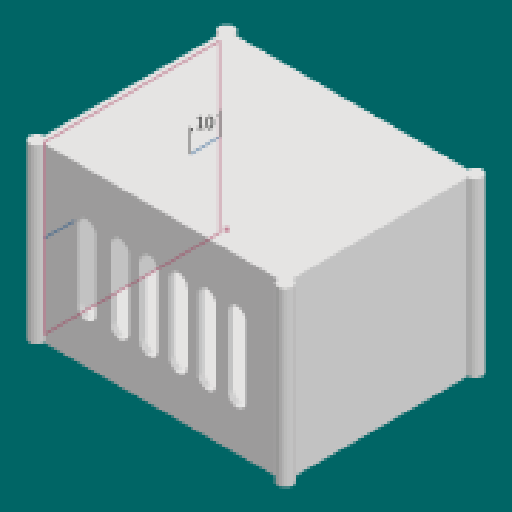
# Autodesk Inventor part: Body_Bottom
Saved by Autodesk Inventor 2025.2 (Build 292293000, 293)
## iProperties
Created: 2025-06-02
Part Number: Body_Bottom
Material: Generic
Document SubType Name: Modeling
Designer: ia088
Density: 1 g/cm^3
Appearance: Default
Author: ia088
Autodesk Inventor part; units mm, degrees
ref_plane "YZ Plane" through (0, 0, 0) normal (1, 0, 0) x (0, 1, 0)
ref_plane "XZ Plane" through (0, 0, 0) normal (0, 1, 0) x (-1, 0, 0)
ref_plane "XY Plane" through (0, 0, 0) normal (0, 0, 1) x (1, 0, 0)
sketch "Sketch1" plane through (0, 0, 0) normal (0, 1, 0) x (-1, 0, 0)
  line L0 (0, 0) -> (-85, 0)
  line L1 (-85, 0) -> (-85, 65)
  line L2 (-85, 65) -> (0, 65)
  line L3 (0, 65) -> (0, 0)
  line L4 (-4, 2) -> (-81, 2)
  line L5 (-83, 4) -> (-83, 61)
  line L6 (-81, 63) -> (-4, 63)
  line L7 (-2, 61) -> (-2, 4)
  circle A0 centre (0, 0) radius 2.5
  circle A1 centre (0, 65) radius 2.5
  circle A2 centre (-85, 65) radius 2.5
  circle A3 centre (-85, 0) radius 2.5
  arc A4 (-4, 2) -> (-2, 4) centre (-4, 4) ccw
  arc A5 (-83, 4) -> (-81, 2) centre (-81, 4) ccw
  arc A6 (-81, 63) -> (-83, 61) centre (-81, 61) ccw
  arc A7 (-2, 61) -> (-4, 63) centre (-4, 61) ccw
  point P0 (0, 62.5)
  point P1 (-2.5, 65)
  point P2 (-82.5, 65)
  point P3 (-85, 62.5)
  point P4 (-85, 2.5)
  point P5 (-82.5, 0)
  point P6 (-2.5, 0)
  point P7 (0, 2.5)
  dimension "d0" = 85
  dimension "d1" = 65
  dimension "d14" = 5
  dimension "d15" = 5
  dimension "d16" = 5
  dimension "d17" = 5
  dimension "d18" = 2
  constraints: 16 end point, 8 centre point, 8 point on circle, 8 tangent, 4 coincident, 4 parallel, 3 equal radius, 2 horizontal, 2 perpendicular
  measures "d0" distance of L1.end L2.end
  measures "d1" distance of L0.end L1.end
  measures "d14" diameter of A0
  measures "d15" diameter of A1
  measures "d16" diameter of A2
  measures "d17" diameter of A3
  measures "d18" radius of A4
extrude "Extrusion1" add sketch "Sketch1" along normal blind 2 contours A3 L1 L0 | A3 L1 A2 L2 A1 L3 A0 L0 | L0 L1 A3 | A0 L3 L0 | L0 L3 A0 | A2 L2 L1 | L1 L2 A2 | A1 L2 L3 | L3 L2 A1 | L4 A5 L5 A6 L6 A7 L7 A4
sketch "Sketch2" plane through (0, 2, 0) normal (0, 1, 0) x (1, 0, 0)
  line L0 (2.5, -65) -> (82.5, -65) projected
  arc A0 (82.5, -65) -> (85, -62.5) centre (85, -65) ccw projected
  line L1 (85, -62.5) -> (85, -2.5) projected
  arc A1 (85, -2.5) -> (82.5, 0) centre (85, 0) ccw projected
  line L2 (82.5, 0) -> (2.5, 0) projected
  arc A2 (2.5, 0) -> (0, -2.5) centre (0, 0) ccw projected
  line L3 (0, -2.5) -> (0, -62.5) projected
  arc A3 (0, -62.5) -> (2.5, -65) centre (0, -65) ccw projected
  line L4 (81, -2) -> (4, -2)
  line L5 (2, -4) -> (2, -61)
  line L6 (4, -63) -> (81, -63)
  line L7 (83, -61) -> (83, -4)
  arc A4 (2, -61) -> (4, -63) centre (4, -61) ccw
  arc A5 (4, -2) -> (2, -4) centre (4, -4) ccw
  arc A6 (81, -63) -> (83, -61) centre (81, -61) ccw
  arc A7 (83, -4) -> (81, -2) centre (81, -4) ccw
  dimension "d25" = 2
  constraints: 8 end point, 8 point on circle, 8 tangent, 4 centre point, 3 equal radius, 2 parallel, 1 horizontal, 1 perpendicular
  measures "d25" radius of A4
extrude "Extrusion2" add sketch "Sketch2" along normal blind 55
sketch "Sketch3" plane through (2.5, 0, 65) normal (0, 0, 1) x (1, 0, 0)
  line L0 (11.33, 17.0347) -> (11.33, 40.7227)
  line L1 (17.642, 40.7227) -> (17.642, 17.0347)
  arc A0 (11.33, 17.0347) -> (17.642, 17.0347) centre (14.486, 17.0347) ccw
  arc A1 (17.642, 40.7227) -> (11.33, 40.7227) centre (14.486, 40.7227) ccw
  line L2 (22.6667, 17.0347) -> (22.6667, 40.7227)
  line L3 (28.9787, 40.7227) -> (28.9787, 17.0347)
  arc A2 (22.6667, 17.0347) -> (28.9787, 17.0347) centre (25.8227, 17.0347) ccw
  arc A3 (28.9787, 40.7227) -> (22.6667, 40.7227) centre (25.8227, 40.7227) ccw
  line L4 (32.7043, 17.0347) -> (32.7043, 40.7227)
  line L5 (39.0162, 40.7227) -> (39.0162, 17.0347)
  arc A4 (32.7043, 17.0347) -> (39.0162, 17.0347) centre (35.8602, 17.0347) ccw
  arc A5 (39.0162, 40.7227) -> (32.7043, 40.7227) centre (35.8602, 40.7227) ccw
  line L6 (42.6524, 17.0347) -> (42.6524, 40.7227)
  line L7 (48.9644, 40.7227) -> (48.9644, 17.0347)
  arc A6 (42.6524, 17.0347) -> (48.9644, 17.0347) centre (45.8084, 17.0347) ccw
  arc A7 (48.9644, 40.7227) -> (42.6524, 40.7227) centre (45.8084, 40.7227) ccw
  line L8 (52.6006, 17.0347) -> (52.6006, 40.7227)
  line L9 (58.9125, 40.7227) -> (58.9125, 17.0347)
  arc A8 (52.6006, 17.0347) -> (58.9125, 17.0347) centre (55.7565, 17.0347) ccw
  arc A9 (58.9125, 40.7227) -> (52.6006, 40.7227) centre (55.7565, 40.7227) ccw
  line L10 (62.7271, 17.0347) -> (62.7271, 40.7227)
  line L11 (69.039, 40.7227) -> (69.039, 17.0347)
  arc A10 (62.7271, 17.0347) -> (69.039, 17.0347) centre (65.8831, 17.0347) ccw
  arc A11 (69.039, 40.7227) -> (62.7271, 40.7227) centre (65.8831, 40.7227) ccw
  point P0 (-2.5, 0)
  point P1 (14.486, 28.8787)
  point P2 (25.8227, 28.8787)
  point P3 (35.8602, 28.8787)
  point P4 (45.8084, 28.8787)
  point P5 (55.7565, 28.8787)
  point P6 (65.8831, 28.8787)
  constraints: 24 end point, 24 point on circle, 24 tangent, 12 centre point, 6 parallel
extrude "Extrusion3" cut sketch "Sketch3" against normal blind 70
sketch "Sketch4" plane through (0, 0, 2.5) normal (-1, 0, 0) x (0, 0, 1)
  line L0 (0, 0) -> (60, 0) projected
  line L1 (60, 0) -> (60, 57) projected
  line L2 (0, 57) -> (60, 57) projected
  line L3 (0, 0) -> (0, 57) projected
  line L4 (0, 28.5) -> (10, 28.5)
  line L5 (60, 28.5) -> (49.7848, 28.5)
  point P0 (-2.5, 0)
  dimension "d44" = 10
  constraints: 4 end point, 2 horizontal, 2 midpoint
  measures "d44" distance of L4.start L4.end
sketch "Sketch6" plane through (0, 57, 0) normal (0, 1, 0) x (1, 0, 0)
  arc A0 (0, -62.5) -> (2.5, -65) centre (0, -65) ccw projected
  line L0 (81, -63) -> (4, -63) projected
  line L1 (2, -61) -> (2, -4) projected
  circle A1 centre (0, -65) radius 1.5
  line L2 (45.4192, -32.5) -> (-3.1549, -32.5)
  circle A2 centre (0, 0) radius 1.5
  circle A3 centre (85, -65) radius 1.5
  circle A4 centre (85, 0) radius 1.5
  dimension "d45" = 3
  dimension "d48" = 65
  dimension "d51" = 85
  constraints: 4 centre point, 2 end point, 2 horizontal, 1 coincident, 1 vertical, 6 other
  measures "d45" diameter of A1
  measures "d48" distance of A1.centre A2.centre
  measures "d51" distance of A1.centre A3.centre
extrude "Extrusion4" cut sketch "Sketch6" against normal blind 10
body "Solid1"
